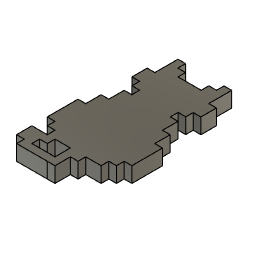
cat_keychain_v1 (Autodesk Fusion 360 design; units mm, degrees)
Autodesk Fusion 360 part; units mm, degrees
sketch "pisica" plane through (0, 0, 0) normal (0, 0, 1) x (1, 0, 0)
  line L0 (-20, 0) -> (-20, 5)
  line L1 (-20, 5) -> (-25, 5)
  line L2 (-25, 5) -> (-25, 10)
  line L3 (-25, 10) -> (-30, 10)
  line L4 (-30, 10) -> (-30, 30)
  line L5 (-30, 30) -> (-25, 30)
  line L6 (-25, 30) -> (-25, 40)
  line L7 (-25, 40) -> (-20, 40)
  line L8 (-20, 40) -> (-20, 50)
  line L9 (-20, 50) -> (-15, 50)
  line L10 (-15, 50) -> (-15, 55.0559)
  line L11 (-15, 55.0559) -> (-20, 55.0559)
  line L12 (-20, 55.0559) -> (-20, 60.1063)
  line L13 (-20, 60.1063) -> (-25, 60.1063)
  line L14 (-25, 60.1063) -> (-25, 69.9795)
  line L15 (-25, 69.9795) -> (-20, 69.9795)
  line L16 (-20, 69.9795) -> (-20, 84.9892)
  line L17 (-20, 84.9892) -> (-15, 84.9892)
  line L18 (-15, 84.9892) -> (-15, 79.9554)
  line L19 (-15, 79.9554) -> (-10, 79.9554)
  line L20 (-10, 79.9554) -> (-10, 75.0569)
  line L21 (-10, 75.0569) -> (5, 75.0569)
  line L22 (5, 75.0569) -> (5, 80.0569)
  line L23 (5, 80.0569) -> (10, 80.0569)
  line L24 (10, 80.0569) -> (10, 84.9215)
  line L25 (10, 84.9215) -> (15, 84.9215)
  line L26 (15, 84.9215) -> (15, 80)
  line L27 (15, 80) -> (15, 70.0231)
  line L28 (15, 70.0231) -> (20, 70.0231)
  line L29 (20, 70.0231) -> (20, 59.9045)
  line L30 (20, 59.9045) -> (15, 59.9045)
  line L31 (15, 59.9045) -> (15, 55.0559)
  line L32 (15, 55.0559) -> (10, 55.0559)
  line L33 (10, 55.0559) -> (10, 50.019)
  line L34 (10, 50.019) -> (15, 50.019)
  line L35 (15, 50.019) -> (15, 50)
  line L36 (15, 50) -> (15, 39.9166)
  line L37 (15, 39.9166) -> (20, 39.9166)
  line L38 (20, 39.9166) -> (20, 29.9166)
  line L39 (20, 29.9166) -> (25, 29.9166)
  line L40 (25, 29.9166) -> (25, 10)
  line L41 (25, 10) -> (20, 10)
  line L42 (20, 10) -> (20, 5)
  line L43 (20, 5) -> (15, 5)
  line L44 (15, 5) -> (15, 0)
  line L45 (15, 0) -> (5, 0)
  line L46 (5, 0) -> (5, -5)
  line L47 (0, -20.0001) -> (0, -20)
  line L48 (-25, -20) -> (-25, -20.0001)
  line L49 (-30, 0) -> (-20, 0)
  line L50 (-10, -10) -> (-5, -10)
  line L51 (-5, -10) -> (-5, -5)
  line L52 (-15, -5) -> (-20, -5)
  line L53 (-5, -15) -> (0, -15)
  line L54 (0, -15) -> (0, -5)
  line L55 (0, -5) -> (5, -5)
  line L56 (-15, 0) -> (-15, -5)
  line L57 (-5, 0) -> (-5, -5)
  line L58 (-20, -5) -> (-20, -10)
  line L59 (-20, -10) -> (-10, -10)
  line L60 (-25, -15) -> (-5, -15)
  line L61 (-25, -10) -> (-25, -15)
  line L62 (-25, -10) -> (-30, -10)
  line L63 (-30, 0) -> (-30, -10)
  line L64 (-15, 0) -> (-5, 0)
  dimension "d5" = 20
  dimension "d6" = 10
  dimension "d7" = 10
  dimension "d8" = 10
  dimension "d9" = 99.9892
  constraint perpendicular L0 L1
  constraint perpendicular L1 L2
  constraint perpendicular L2 L3
  constraint perpendicular L3 L4
  constraint perpendicular L4 L5
  constraint perpendicular L5 L6
  constraint perpendicular L6 L7
  constraint perpendicular L7 L8
  constraint perpendicular L8 L9
  constraint perpendicular L9 L10
  constraint perpendicular L10 L11
  constraint perpendicular L11 L12
  constraint perpendicular L12 L13
  constraint perpendicular L13 L14
  constraint perpendicular L14 L15
  constraint perpendicular L15 L16
  constraint perpendicular L4 L17
  constraint perpendicular L11 L18
  constraint perpendicular L18 L19
  constraint perpendicular L19 L20
  constraint perpendicular L20 L21
  constraint perpendicular L21 L22
  constraint perpendicular L22 L23
  constraint perpendicular L21 L24
  constraint perpendicular L24 L25
  constraint perpendicular L25 L26
  constraint perpendicular L25 L27
  constraint perpendicular L27 L28
  constraint perpendicular L28 L29
  constraint perpendicular L29 L30
  constraint perpendicular L30 L31
  constraint perpendicular L31 L32
  constraint perpendicular L30 L33
  constraint perpendicular L4 L34
  constraint perpendicular L34 L35
  constraint perpendicular L34 L36
  constraint perpendicular L36 L37
  constraint perpendicular L34 L38
  constraint perpendicular L38 L39
  constraint perpendicular L39 L40
  constraint perpendicular L40 L41
  constraint perpendicular L41 L42
  constraint perpendicular L42 L43
  constraint perpendicular L43 L44
  constraint perpendicular L44 L45
  constraint perpendicular L45 L46
  constraint perpendicular L50 L51
  constraint perpendicular L51 L52
  constraint perpendicular L53 L54
  constraint vertical L56
  constraint perpendicular L52 L57
  constraint perpendicular L58 L59
  constraint perpendicular L60 L61
  constraint perpendicular L62 L63
  constraint perpendicular L57 L64
  measures "d5" distance of L3 L5
  measures "d6" distance of L5 L7
  measures "d7" distance of L37 L39
  measures "d8" distance of L7 L9
  measures "d9" distance of L17 L53
extrude "Extrude1" add sketch "pisica" along normal blind 10
named bodies: "breloc_pisica"
